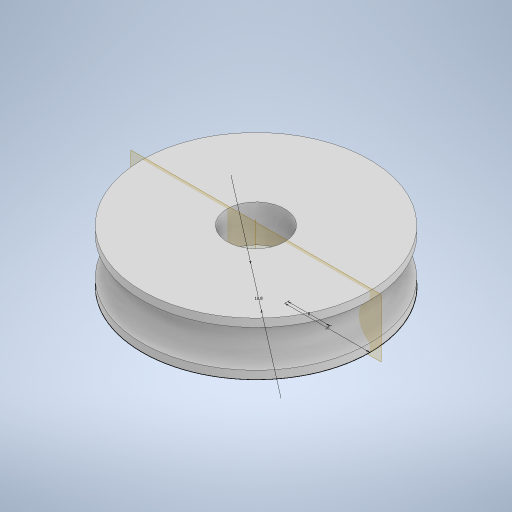
# Autodesk Inventor part: 코일건원통꼽게1
Saved by Autodesk Inventor 2023 (Build 270158000, 158)
## iProperties
Created: 2023-04-25
Part Number: 코일건원통꼽게1
Material: 일반
Document SubType Name: Modeling
Designer: rlatk
Density: 1 g/cm^3
Appearance: 기본값
Author: rlatk
Autodesk Inventor part; units mm, degrees
ref_plane "YZ Plane" through (0, 0, 0) normal (1, 0, 0) x (0, 1, 0)
ref_plane "XZ Plane" through (0, 0, 0) normal (0, 1, 0) x (-1, 0, 0)
sketch "스케치1" plane through (0, 0, 0) normal (0, 1, 0) x (-1, 0, 0)
  circle A0 centre (0, 0) radius 5.4
  circle A1 centre (0, 0) radius 21.4
  circle A2 centre (0, 0) radius 13.4
  dimension "d0" = 10.8
  dimension "d1" = 16
  dimension "d8" = 8
  constraints: 3 centre point, 1 coincident
  measures "d0" diameter of A0
  measures "d1" radial gap between concentric circles of A0 A1
  measures "d8" radial gap between concentric circles of A0 A2
extrude "돌출1" add sketch "스케치1" along normal blind 10 contours A1 | A2
sketch "스케치2" plane through (0, 0, 0) normal (0, 0, 1) x (1, 0, 0)
  line L0 (-21.4, 0) -> (-21.4, 10) projected
  arc A0 (-21.4, 1.5) -> (-21.4355, 8.5) centre (-23.3541, 4.9902) ccw
  line L1 (0, -2) -> (0, 12) projected
  point P0 (0, 0)
  point P1 (-21.4, 8.4804)
  dimension "d4" = 4
  dimension "d5" = 1.5
  dimension "d6" = 1.5
  constraints: 2 point on circle, 1 centre point, 1 point on line
  measures "d4" radius of A0
  measures "d5" vertical distance of L0.end A0.end
  measures "d6" distance of L0.start A0.start
revolve "회전1" cut sketch "스케치2" angle 360 about axis through (0, -10, 0) along (0, 1, 0)
extrude "돌출2" cut sketch "스케치1" along normal blind 3 contours A2
